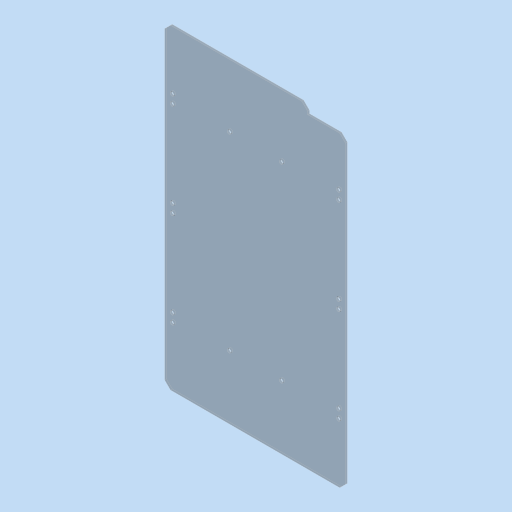
# Autodesk Inventor part: enc-BackPanel Mitte
Saved by Autodesk Inventor 2023.2 (Build 272271000, 271)
## iProperties
Created: 2023-12-04
Part Number: enc-BackPanel Mitte
Material: Generisch
Document SubType Name: Modeling
Designer: Nils Bade
Density: 1 g/cm^3
Appearance: PVC Verglasung
Author: Nils Bade
Autodesk Inventor part; units mm, degrees
ref_plane "YZ Plane" through (0, 0, 0) normal (1, 0, 0) x (0, 1, 0)
ref_plane "XZ Plane" through (0, 0, 0) normal (0, 1, 0) x (-1, 0, 0)
ref_plane "XY Plane" through (0, 0, 0) normal (0, 0, 1) x (1, 0, 0)
sketch "Skizze1" plane through (0, 0, 0) normal (0, 0, 1) x (1, 0, 0)
  line L0 (-155, 270.5) -> (155, 270.5)
  line L1 (155, 270.5) -> (155, -270.5)
  line L2 (155, -270.5) -> (-155, -270.5)
  line L3 (-155, -270.5) -> (-155, 270.5)
  line L4 (-155, 270.5) -> (155, -270.5) construction
  line L5 (155, 270.5) -> (-155, -270.5) construction
  line L6 (-77.5, 270.5) -> (-77.5, -270.5) construction
  line L7 (0, 396.7) -> (0, -381.7) construction
  line L8 (-142.5, 270.5) -> (-142.5, -270.5) construction
  line L9 (-155, -162.3) -> (155, -162.3) construction
  circle A0 centre (-142.5, -154.8) radius 3.25
  circle A1 centre (-142.5, -169.8) radius 3.25
  line L10 (-230, 0) -> (295, 0) construction
  circle A2 centre (-142.5, 7.5) radius 3.25
  circle A3 centre (-142.5, -7.5) radius 3.25
  circle A4 centre (-142.5, 154.8) radius 3.25
  circle A5 centre (-142.5, 169.8) radius 3.25
  circle A6 centre (142.5, -154.8) radius 3.25
  circle A7 centre (142.5, -169.8) radius 3.25
  circle A8 centre (142.5, 7.5) radius 3.25
  circle A9 centre (142.5, -7.5) radius 3.25
  circle A10 centre (142.5, 169.8) radius 3.25
  circle A11 centre (142.5, 154.8) radius 3.25
  circle A12 centre (-44.5, -162.3) radius 3.25
  circle A13 centre (44.5, -162.3) radius 3.25
  circle A14 centre (-44.5, 162.3) radius 3.25
  circle A15 centre (44.5, 162.3) radius 3.25
  line L11 (220, 285.5) -> (90, 285.5) construction
  line L12 (90, 285.5) -> (90, 255.5)
  line L13 (90, 255.5) -> (220, 255.5)
  line L14 (220, 255.5) -> (220, 285.5) construction
  line L15 (220, 285.5) -> (90, 255.5) construction
  line L16 (90, 285.5) -> (220, 255.5) construction
  point P0 (0, 0)
  point P1 (155, 255.5)
  point P2 (90, 270.5)
  dimension "d0" = 541
  dimension "d1" = 310
  dimension "d2" = 77.5
  dimension "d3" = 12.5
  dimension "d4" = 108.2
  dimension "d5" = 6.5
  dimension "d6" = 7.5
  dimension "d7" = 6.5
  dimension "d8" = 7.5
  dimension "d9" = 7.5
  dimension "d10" = 6.5
  dimension "d11" = 6.5
  dimension "d12" = 44.5
  dimension "d15" = 130
  dimension "d16" = 15
  constraints: 30 end point, 16 centre point, 12 symmetric about line, 8 point on line, 4 midpoint, 4 parallel, 4 perpendicular, 2 horizontal, 1 vertical, 12 other
  measures "d0" distance of L0.end L1.end
  measures "d1" distance of L1.end L2.end
  measures "d2" distance between parallel lines of L3 L6
  measures "d3" distance between parallel lines of L3 L8
  measures "d4" distance between parallel lines of L2 L9
  measures "d5" diameter of A0
  measures "d6" distance from line of L9 A0.centre
  measures "d7" diameter of A2
  measures "d8" distance from line of L10 A2.centre
  measures "d9" distance from line of L10 A3.centre
  measures "d10" diameter of A3
  measures "d11" diameter of A12
  measures "d12" distance from line of L7 A12.centre
  measures "d15" distance of L11.start L11.end
  measures "d16" distance between parallel lines of L0 L13
extrude "Extrusion1" add sketch "Skizze1" along normal blind 3 contours L0 L12 L13 L1 L2 L3
chamfer "Fase1" distance 10 angle 45 5 edges at (90, 270.5, 1.5) (155, 255.5, 1.5) (155, -270.5, 1.5) (-155, -270.5, 1.5) (-155, 270.5, 1.5)
equation "\"d2\" = 0.25 * d1"
equation "\"d4\" = 0.2 * d0"
equation "\"d7\" = d5"
equation "\"d8\" = d6"
equation "\"d9\" = d6"
equation "\"d10\" = d5"
